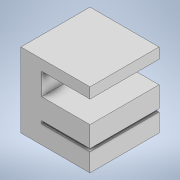
# Autodesk Inventor part: base
Saved by Autodesk Inventor 2020 (Build 240168000, 168)
## iProperties
Created: 2021-01-27
Part Number: base
Material: Generic
Document SubType Name: Modeling
Designer: pduy110
Density: 1 g/cm^3
Appearance: Default
Author: pduy110
Autodesk Inventor part; units mm, degrees
ref_plane "YZ Plane" through (0, 0, 0) normal (1, 0, 0) x (0, 1, 0)
ref_plane "XZ Plane" through (0, 0, 0) normal (0, 1, 0) x (-1, 0, 0)
ref_plane "XY Plane" through (0, 0, 0) normal (0, 0, 1) x (1, 0, 0)
sketch "Sketch1" plane through (0, 0, 0) normal (0, 0, 1) x (1, 0, 0)
  line L0 (0, 27) -> (0, -27)
  line L1 (0, -27) -> (50, -27)
  line L2 (50, -27) -> (50, -13.7241)
  line L3 (50, -13.7241) -> (15, -13.7241)
  line L4 (15, -13.7241) -> (15, -11.7241)
  line L5 (15, -11.7241) -> (50, -11.7241)
  line L6 (50, -11.7241) -> (50, 3.2759)
  line L7 (50, 3.2759) -> (15, 3.2759)
  line L8 (15, 3.2759) -> (15, 19.2759)
  line L9 (15, 19.2759) -> (50, 19.2759)
  line L10 (50, 19.2759) -> (50, 27)
  line L11 (50, 27) -> (0, 27)
  point P0 (0, 0)
  point P1 (0, 0)
  point P2 (0, 0)
  dimension "d0" = 15
  dimension "d1" = 16
  dimension "d2" = 2
  dimension "d3" = 50
  dimension "d4" = 54
  dimension "d7" = 15
  constraints: 24 end point, 8 perpendicular, 6 point on line, 2 coincident, 1 midpoint, 1 vertical
  measures "d0" distance between parallel lines of L5 L7
  measures "d1" distance between parallel lines of L7 L9
  measures "d2" distance between parallel lines of L3 L5
  measures "d3" distance between parallel lines of L2 L0
  measures "d4" distance between parallel lines of L1 L11
  measures "d7" distance between parallel lines of L8 L0
extrude "Extrusion1" add sketch "Sketch1" along normal blind 50
equation "\"d0\" = aluminium_gap_distance"
equation "\"d1\" = acrylic_total_thickness"
equation "\"d2\" = aluminium_thickness"
equation "\"aluminium_gap_distance\" = 15"
equation "\"acrylic_total_thickness\" = 16"
equation "\"aluminium_thickness\" = 2"
body "Solid1"
